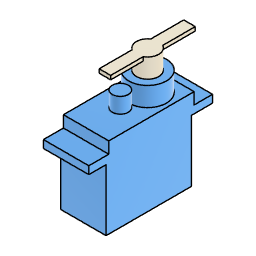
Serwo (Autodesk Fusion 360 design; units mm, degrees)
part number: 2025-03-31-19-35-40-270
Autodesk Fusion 360 part; units mm, degrees
sketch "Szkic1" plane through (0, 0, 0) normal (0, 0, 1) x (1, 0, 0)
  line L0 (5, 5.5) -> (-6.8, 5.5)
  line L1 (-6.8, 5.5) -> (-6.8, -16.7)
  line L2 (-6.8, -16.7) -> (5, -16.7)
  line L3 (5, -16.7) -> (5, 5.5)
  dimension "d5" = 11.8
  dimension "d6" = 22.2
  constraint horizontal L0
  constraint vertical L1
  constraint horizontal L2
  constraint vertical L3
  measures "d5" distance of L0.start L0.end
  measures "d6" distance of L0.start L2.end
extrude "Wyciągnięcie proste1" add sketch "Szkic1" along normal blind 16 makes body 1
sketch "Szkic2" plane through (0, 0, 16) normal (0, 0, 1) x (-1, 0, 0)
  line L0 (-5, 16.7) -> (-5, -5.5)
  line L1 (-5, -5.5) -> (6.8, -5.5)
  line L2 (6.8, -5.5) -> (6.8, 16.7)
  line L3 (6.8, 16.7) -> (-5, 16.7)
  line L4 (-5, -11) -> (6.8, -11)
  line L5 (6.8, -11) -> (6.8, 21.2)
  line L6 (6.8, 21.2) -> (-5, 21.2)
  line L7 (-5, 21.2) -> (-5, -11)
  dimension "d9" = 11.8
  dimension "d10" = 32.2
  constraint horizontal L4
  constraint vertical L5
  constraint horizontal L6
  constraint vertical L7
  measures "d9" distance of L4.start L4.end
  measures "d10" distance of L4.start L6.end
extrude "Wyciągnięcie proste2" add sketch "Szkic2" along normal blind 2 bodies 1
sketch "Szkic3" plane through (0, 0, 18) normal (0, 0, 1) x (-1, 0, 0)
  line L0 (-5, 21.2) -> (-5, -11)
  line L1 (-5, -11) -> (6.8, -11)
  line L2 (6.8, -11) -> (6.8, 21.2)
  line L3 (6.8, 21.2) -> (-5, 21.2)
  line L4 (-5, 16) -> (6.8, 16)
  line L5 (6.8, 16) -> (6.8, -6.2)
  line L6 (6.8, -6.2) -> (-5, -6.2)
  line L7 (-5, -6.2) -> (-5, 16)
  dimension "d13" = 11.8
  dimension "d14" = 22.2
  constraint horizontal L4
  constraint vertical L5
  constraint horizontal L6
  constraint vertical L7
  constraint coincident L0 L4.start
  measures "d13" distance of L4.start L4.end
  measures "d14" distance of L4.start L6.end
extrude "Wyciągnięcie proste3" add sketch "Szkic3" along normal blind 3 contours L0 L2 L4 L5 L6 L7 bodies 1
sketch "Szkic4" plane through (0, 0, 21) normal (0, 0, 1) x (-1, 0, 0)
  line L0 (-5, -6.2) -> (6.8, -6.2)
  line L1 (6.8, -6.2) -> (6.8, 16)
  line L2 (6.8, 16) -> (-5, 16)
  line L3 (-5, 16) -> (-5, -6.2)
  circle A0 centre (0.9, 0) radius 4.9
  circle A1 centre (1, 7) radius 2.1007
  constraint tangent A0 A1
extrude "Wyciągnięcie proste4" add sketch "Szkic4" along normal blind 5 contours A0 bodies 1
extrude "Wyciągnięcie proste5" add sketch "Szkic4" along normal blind 4 contours A1 bodies 1
sketch "Szkic5" plane through (0, 0, 26) normal (0, 0, 1) x (-1, 0, 0)
  circle A0 centre (0.9, 0) radius 4.9
  circle A1 centre (0.9, 0) radius 2.9
  constraint concentric A0 A1
extrude "Wyciągnięcie proste6" add sketch "Szkic5" along normal blind 5 separate body contours A1 makes body 2
sketch "Szkic6" plane through (0, 0, 0) normal (0, 1, 0) x (1, 0, 0)
  line L0 (-2.5, -31) -> (0.5, -31)
  line L1 (0.5, -31) -> (0.5, -30)
  line L2 (0.5, -30) -> (-2.5, -30)
  line L3 (-2.5, -30) -> (-2.5, -31)
  line L4 (-2.5, -31) -> (0.5, -30) construction
  line L5 (0.5, -31) -> (-2.5, -30) construction
  point P0 (-1, -30.5)
  constraint horizontal L0
  constraint perpendicular L0 L1
  constraint parallel L0 L2
  constraint parallel L1 L3
  constraint coincident L4 P0
  constraint coincident L5 P0
extrude "Wyciągnięcie proste7" add sketch "Szkic6" along normal blind 11 and the other way blind 11 bodies 2
named bodies: "servo_base", "servo_smiglo"
